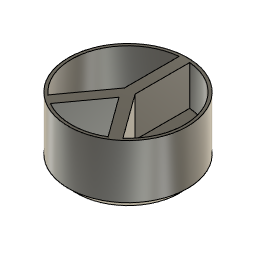
led-lamp-cap (Autodesk Fusion 360 design; units mm, degrees)
Autodesk Fusion 360 part; units mm, degrees
sketch "Sketch1" plane through (0, 0, 0) normal (0, 0, 1) x (1, 0, 0)
  line L0 (-1.875, 0.6092) -> (-1.875, 19.5)
  line L1 (-1.875, 19.5) -> (1.875, 19.5)
  line L2 (1.875, 19.5) -> (1.875, 0.6092)
  line L3 (1.875, 0.6092) -> (12.9787, -14.6737)
  line L4 (12.9787, -14.6737) -> (9.9449, -16.8779)
  line L5 (9.9449, -16.8779) -> (0, -3.1899)
  line L6 (0, -3.1899) -> (-9.9449, -16.8779)
  line L7 (-9.9449, -16.8779) -> (-12.9787, -14.6737)
  line L8 (-12.9787, -14.6737) -> (-1.875, 0.6092)
  line L9 (0, 0) -> (-11.4618, -15.7758)
  line L10 (11.4618, -15.7758) -> (0, 0)
  line L11 (0, 19.5) -> (0, 0)
  dimension "d4" = 144
  dimension "d5" = 144
  dimension "d6" = 19.5
  dimension "d7" = 3.75
  constraint coincident L9.start L10.end
  constraint midpoint L1 L11.start
  constraint perpendicular L1 L11
  constraint perpendicular L7 L9
  constraint midpoint L7 L9.end
  constraint vertical L11
  constraint parallel L0 L2
  constraint parallel L3 L5
  constraint perpendicular L4 L10
  constraint midpoint L4 L10.start
  constraint parallel L6 L8
  constraint equal L10 L11
  constraint equal L9 L10
  constraint parallel L6 L9
  constraint parallel L5 L10
  constraint parallel L2 L11
  constraint equal L5 L6
  constraint equal L3 L8
  constraint equal L1 L4
  measures "d4" angle of L10 L11
  measures "d5" angle of L9 L11
  measures "d6" distance of L9.start L11.start
  measures "d7" distance of L3.end L4.end
extrude "Extrude1" add sketch "Sketch1" along normal blind 17 makes body 1
sketch "Sketch2" plane through (0, 0, 0) normal (0, 0, -1) x (1, 0, 0)
  line L0 (-9.9449, 16.8779) -> (-12.9787, 14.6737)
  line L1 (-12.9787, 14.6737) -> (-1.875, -0.6092)
  line L2 (-1.875, -0.6092) -> (-1.875, -19.5)
  line L3 (-1.875, -19.5) -> (1.875, -19.5)
  line L4 (1.875, -19.5) -> (1.875, -0.6092)
  line L5 (1.875, -0.6092) -> (12.9787, 14.6737)
  line L6 (12.9787, 14.6737) -> (9.9449, 16.8779)
  line L7 (9.9449, 16.8779) -> (0, 3.1899)
  line L8 (0, 3.1899) -> (-9.9449, 16.8779)
  circle A0 centre (0, 0) radius 17
  circle A1 centre (0, 0) radius 20
  dimension "d16" = 40
  dimension "d17" = 3
  constraint coincident A0.centre A1.centre
  constraint concentric A0 A1
  measures "d16" diameter of A1
  measures "d17" distance of A0 A1
extrude "Extrude2" add sketch "Sketch2" against normal blind 3 separate body contours L7 L8 A0 | L1 L2 A0 | L4 L5 A0 | A1 makes body 2
sketch "Sketch4" plane through (0, 0, 3) normal (0, 0, 1) x (-1, 0, 0)
  line L0 (-1.875, -0.6092) -> (-12.9787, 14.6737)
  line L1 (-12.9787, 14.6737) -> (-9.9449, 16.8779)
  line L2 (-9.9449, 16.8779) -> (0, 3.1899)
  line L3 (0, 3.1899) -> (9.9449, 16.8779)
  line L4 (9.9449, 16.8779) -> (12.9787, 14.6737)
  line L5 (12.9787, 14.6737) -> (1.875, -0.6092)
  line L6 (1.875, -0.6092) -> (1.875, -19.5)
  line L7 (1.875, -19.5) -> (-1.875, -19.5)
  line L8 (-1.875, -19.5) -> (-1.875, -0.6092)
  circle A0 centre (0, 0) radius 20
  line L9 (1.875, -19.5) -> (1.875, -19.9119)
  arc A1 (-1.875, -19.9119) -> (1.875, -19.9119) centre (0, 0) ccw
  line L10 (1.875, -19.5) -> (-1.875, -19.5)
  line L11 (-1.875, -19.5) -> (-1.875, -19.9119)
  constraint vertical L9
  constraint perpendicular L9 L10
  constraint coincident L9.end A1.end
  constraint parallel L9 L11
  constraint coincident L6.end L7.start
  constraint coincident L7.end L8.start
  constraint coincident A0 A1.start
  constraint coincident A0 L9.end
  constraint coincident L11 A1.start
  constraint coincident A1.start L11.end
  constraint coincident A0.centre A1.centre
extrude "Extrude3" add sketch "Sketch4" along normal up to surface (14 mm away) contours L7 A0 L9 A1 L10 L11 bodies 1 2
pattern_circular "C-Pattern1" count 2 over 144 about axis through (0, 0, 1.75) along (0, 0, 1) of "Extrude3"
pattern_circular "C-Pattern2" count 2 over 144 about axis through (0, 0, 1.75) along (0, 0, -1) of "Extrude3"
extrude "Extrude7" add 1 faces at (4.7423, 7.1112, 0) along direction (0, 0, -1) blind 5 on bodies 1 bodies 1
sketch "Sketch8" plane through (0, 0, -5) normal (0, 0, -1) x (1, 0, 0)
  circle A0 centre (0, 0) radius 20
  circle A1 centre (0, 0) radius 21
  dimension "d40" = 42
  constraint coincident A0.centre A1.centre
  measures "d40" diameter of A1
extrude "Extrude8" add sketch "Sketch8" against normal up to surface (22 mm away) bodies 1
chamfer "Chamfer1" distance 3 angle 45 1 edges at (-19.5789, 7.5939, -5) on bodies 1
